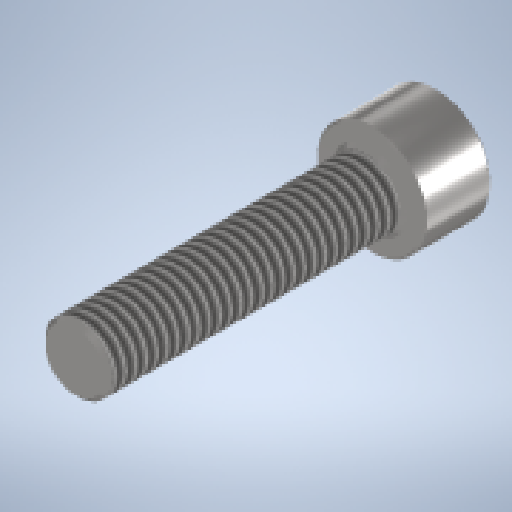
# Autodesk Inventor part: SHCSM8x35
Saved by Autodesk Inventor 2024 (Build 280153000, 153)
## iProperties
Created: 2024-09-05
Part Number: SHCSM8x35
Material: Stainless Steel
Document SubType Name: Modeling
Designer: Ishaan
Density: 8 g/cm^3
Appearance: Semi-Polished
Author: Ishaan
Autodesk Inventor part; units mm, degrees
ref_plane "YZ Plane" through (0, 0, 0) normal (1, 0, 0) x (0, 1, 0)
ref_plane "XZ Plane" through (0, 0, 0) normal (0, 1, 0) x (-1, 0, 0)
ref_plane "XY Plane" through (0, 0, 0) normal (0, 0, 1) x (1, 0, 0)
sketch "Sketch1" plane through (0, 0, 0) normal (0, 0, 1) x (1, 0, 0)
  circle A0 centre (0, 0) radius 6.5
  circle A1 centre (0, 0) radius 4
  dimension "d0" = 13
  dimension "d1" = 8
  constraints: 2 centre point, 2 coincident
  measures "d0" diameter of A0
  measures "d1" diameter of A1
extrude "Extrusion1" add sketch "Sketch1" along normal blind 35 contours A1
extrude "Extrusion2" add sketch "Sketch1" against normal blind 8 contours A0 | A1
thread "Thread1" size "M8x1.25" class "6g" standard "ANSI Metric M Profile" full length
chamfer "Chamfer1" distance 0.25 angle 45 2 edges at (-6.5, 0, 0) (-6.5, 0, -8)
sketch "Sketch2" plane through (0, 0, -8) normal (0, 0, -1) x (-1, 0, 0)
  circle A0 centre (0, 0) radius 2.75
  line L0 (-1.7321, 3) -> (1.7321, 3)
  line L1 (1.7321, 3) -> (3.4641, 0)
  line L2 (3.4641, 0) -> (1.7321, -3)
  line L3 (1.7321, -3) -> (-1.7321, -3)
  line L4 (-1.7321, -3) -> (-3.4641, 0)
  line L5 (-3.4641, 0) -> (-1.7321, 3)
  dimension "d11" = 5.5
  dimension "d12" = 6
  constraints: 12 end point, 2 coincident, 1 centre point, 1 horizontal, 13 other
  measures "d11" diameter of A0
  measures "d12" distance between parallel lines of L3 L0
hole "Hole1" at (0, 0, -8) direction (0, 0, 1) diameter 5.5 depth 4 tip angle 150
chamfer "Chamfer2" distance 1 angle 45 1 edges at (0, -2.75, -8)
extrude "Extrusion4" cut sketch "Sketch2" against normal up to surface contours A0 | L0 L1 L2 L3 L4 L5 round surface about axis through (0, 0, -3.6316) along (0, 0, -1) radius 1.375 half angle 75 far side no
chamfer "Chamfer3" distance 0.5 angle 45 2 edges at (-4, 0, 0) (-4, 0, 35)
equation "\"d23\" = d11"
body "Solid1"
